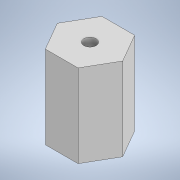
# Autodesk Inventor part: BruteForceCoupler
Saved by Autodesk Inventor 2020.1 (Build 241239000, 239)
## iProperties
Created: 2019-12-05
Part Number: BruteForceCoupler
Material: Generic
Document SubType Name: Modeling
Designer: super
Density: 1 g/cm^3
Appearance: Default
Author: super
Autodesk Inventor part; units mm, degrees
ref_plane "YZ Plane" through (0, 0, 0) normal (1, 0, 0) x (0, 1, 0)
ref_plane "XZ Plane" through (0, 0, 0) normal (0, 1, 0) x (-1, 0, 0)
ref_plane "XY Plane" through (0, 0, 0) normal (0, 0, 1) x (1, 0, 0)
sketch "Sketch1" plane through (0, 0, 0) normal (0, 1, 0) x (-1, 0, 0)
  line L0 (6.7, 0) -> (3.35, -5.8024)
  line L1 (3.35, -5.8024) -> (-3.35, -5.8024)
  line L2 (-3.35, -5.8024) -> (-6.7, 0)
  line L3 (-6.7, 0) -> (-3.35, 5.8024)
  line L4 (-3.35, 5.8024) -> (3.35, 5.8024)
  line L5 (3.35, 5.8024) -> (6.7, 0)
  point P0 (0, 0)
  dimension "d1" = 6.7
  constraints: 12 end point, 2 parallel, 1 horizontal
  measures "d1" distance of L0.start L0.end
extrude "Extrusion1" add sketch "Sketch1" along normal blind 17
sketch "Sketch2" plane through (0, 17, 0) normal (0, 1, 0) x (1, 0, 0)
  circle A0 centre (0, 0) radius 1.25
  dimension "d4" = 2.5
  constraints: 1 centre point, 1 coincident
  measures "d4" diameter of A0
extrude "Extrusion2" cut sketch "Sketch2" against normal blind 10
body "Solid1"
